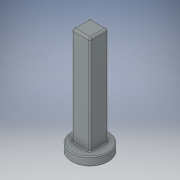
# Autodesk Inventor part: AXp2c
Saved by Autodesk Inventor 2019.3 (Build 233278000, 278)
## iProperties
Company: Unknown
Created: 2018-11-05
Part Number: AXp2c
Material: Generic
Description: Unknown
Document SubType Name: Modeling
Designer: Varga Daniel
Density: 1 g/cm^3
Appearance: Default
Sending System: DEX
Preprocessor: ST-DEVELOPER v16.7
Axle_length: 20,000 mm
Upper_fillet: 0,400 mm
Title: Axeis 2
Author: Unknown
Autodesk Inventor part; units mm, degrees
ref_plane "YZ Plane" through (0, 0, 0) normal (1, 0, 0) x (0, 1, 0)
ref_plane "XZ Plane" through (0, 0, 0) normal (0, 1, 0) x (-1, 0, 0)
ref_plane "XY Plane" through (0, 0, 0) normal (0, 0, 1) x (1, 0, 0)
derived "Connector_pin_base.ipt"
sketch "Pin_base_sketch" plane through (0, 0, 0) normal (0, 0, 1) x (1, 0, 0)
  line L0 (0, 0) -> (23.0918, 0) construction
  line L1 (0, 0) -> (0, 6.22) construction
  line L2 (0, 3.75) -> (0.563, 3.75)
  line L3 (0.863, 3.45) -> (0.863, 2.475)
  line L4 (0.863, 2.475) -> (9.988, 2.475)
  line L5 (9.988, 2.475) -> (9.988, 0)
  line L6 (0, 0) -> (0, 3.75)
  line L7 (0, 0) -> (9.988, 0)
  line L8 (9.288, 2.475) -> (9.288, 2.6)
  line L9 (9.988, 2.475) -> (9.988, 2.4774)
  arc A0 (9.988, 2.4774) -> (9.8454, 2.7031) centre (9.738, 2.4774) ccw
  arc A1 (9.8454, 2.7031) -> (9.288, 2.6) centre (9.6379, 2.267) ccw
  line L10 (9.8454, 2.7031) -> (9.8454, -0.0362) construction
  line L11 (8.9584, 2.75) -> (10.3858, 2.75) construction
  arc A2 (0.863, 3.45) -> (0.563, 3.75) centre (0.563, 3.45) ccw
  line L12 (0.863, 2.475) -> (0.863, 0)
  line L13 (-0.863, 2.475) -> (-0.863, 0)
  line L14 (-0.863, 3.45) -> (-0.863, 2.475)
  arc A3 (-0.563, 3.75) -> (-0.863, 3.45) centre (-0.563, 3.45) ccw
  line L15 (0, 3.75) -> (-0.563, 3.75)
  line L16 (0, 0) -> (-23.0918, 0) construction
  line L17 (0, 0) -> (-9.988, 0)
  line L18 (-0.863, 2.475) -> (-9.988, 2.475)
  line L19 (-9.288, 2.475) -> (-9.288, 2.6)
  arc A4 (-9.288, 2.6) -> (-9.8454, 2.7031) centre (-9.6379, 2.267) ccw
  arc A5 (-9.8454, 2.7031) -> (-9.988, 2.4774) centre (-9.738, 2.4774) ccw
  line L20 (-9.988, 2.475) -> (-9.988, 2.4774)
  line L21 (-8.9584, 2.75) -> (-10.3858, 2.75) construction
  line L22 (-9.8454, 2.7031) -> (-9.8454, -0.0362) construction
  line L23 (-9.988, 2.475) -> (-9.988, 0)
  line L24 (9.638, 3.1946) -> (9.638, -1.2485) construction
derived "Base_part.ipt"
sketch "Axle_sketch" plane through (0, 0, 0) normal (0, 1, 0) x (-1, 0, 0)
  circle A0 centre (-15.8957, 4.3197) radius 2.5 construction
  line L0 (-14.4207, 2.4447) -> (-17.3707, 2.4447)
  line L1 (-17.7707, 2.8447) -> (-17.7707, 5.7947)
  line L2 (-17.3707, 6.1947) -> (-14.4207, 6.1947)
  line L3 (-14.0207, 5.7947) -> (-14.0207, 2.8447)
  line L4 (-14.0207, 2.4447) -> (-17.7707, 6.1947) construction
  line L5 (-17.7707, 2.4447) -> (-14.0207, 6.1947) construction
  arc A1 (-14.4207, 2.4447) -> (-14.0207, 2.8447) centre (-14.4207, 2.8447) ccw
  arc A2 (-17.7707, 2.8447) -> (-17.3707, 2.4447) centre (-17.3707, 2.8447) ccw
  arc A3 (-14.0207, 5.7947) -> (-14.4207, 6.1947) centre (-14.4207, 5.7947) ccw
  arc A4 (-17.3707, 6.1947) -> (-17.7707, 5.7947) centre (-17.3707, 5.7947) ccw
  point P0 (0, 0)
sketch "Sketch1" plane through (0, 0, 0) normal (0, 1, 0) x (-1, 0, 0)
  line L0 (-1.475, -1.875) -> (1.475, -1.875)
  line L1 (1.875, -1.475) -> (1.875, 1.475)
  line L2 (1.475, 1.875) -> (-1.475, 1.875)
  line L3 (-1.875, 1.475) -> (-1.875, -1.475)
  line L4 (-1.875, -1.875) -> (1.875, 1.875) construction
  line L5 (1.875, -1.875) -> (-1.875, 1.875) construction
  arc A0 (-1.875, -1.475) -> (-1.475, -1.875) centre (-1.475, -1.475) ccw
  arc A1 (1.475, -1.875) -> (1.875, -1.475) centre (1.475, -1.475) ccw
  arc A2 (1.875, 1.475) -> (1.475, 1.875) centre (1.475, 1.475) ccw
  arc A3 (-1.475, 1.875) -> (-1.875, 1.475) centre (-1.475, 1.475) ccw
  circle A4 centre (0, 0) radius 2.5 construction
  line L6 (-14.4207, 2.4447) -> (-17.3707, 2.4447) construction
  arc A5 (-14.4207, 2.4447) -> (-14.0207, 2.8447) centre (-14.4207, 2.8447) ccw construction
  line L7 (-14.0207, 5.7947) -> (-14.0207, 2.8447) construction
  circle A6 centre (-15.8957, 4.3197) radius 2.5 construction
  line L8 (-17.3707, 6.1947) -> (-14.4207, 6.1947) construction
  arc A7 (-17.3707, 6.1947) -> (-17.7707, 5.7947) centre (-17.3707, 5.7947) ccw construction
  line L9 (-17.7707, 2.8447) -> (-17.7707, 5.7947) construction
  arc A8 (-17.7707, 2.8447) -> (-17.3707, 2.4447) centre (-17.3707, 2.8447) ccw construction
  arc A9 (-14.0207, 5.7947) -> (-14.4207, 6.1947) centre (-14.4207, 5.7947) ccw construction
  dimension "d0" = 3.75
  dimension "d1" = 3.75
  dimension "d2" = 0.4
  dimension "d11" = 5
  dimension "d13" = 3.75
  dimension "d14" = 0.4
  constraints: 12 end point, 8 point on circle, 8 point on line, 8 tangent, 5 centre point, 3 equal radius, 2 midpoint, 2 parallel, 1 coincident, 1 horizontal, 1 perpendicular
  measures "d0" distance of L4.end L5.end
  measures "d1" distance between parallel lines of L2 L0
  measures "d2" radius of A0
  measures "d11" diameter of A4
  measures "d13" distance between parallel lines of L7 L9
  measures "d14" radius of A8
extrude "Extrusion4" add sketch "Sketch1" along normal blind 20
fillet "Fillet2" radius 0.4 8 edges at (1.7578, 20, -1.7578) (0, 20, -1.875) (-1.7578, 20, -1.7578) (-1.875, 20, 0) (-1.7578, 20, 1.7578) (0, 20, 1.875) (1.7578, 20, 1.7578) (1.875, 20, 0)
ref_plane "Work Plane3" through (-1.475, 0, 0) normal (0, 0, 1) x (1, 0, 0)
ref_plane "Work Plane4" through (0, 0, -1.475) normal (-1, 0, 0) x (0, 0, 1)
sketch "Sketch6" plane through (0, 0, 0) normal (0, 0, 1) x (1, 0, 0)
  line L0 (0.863, 2.475) -> (0.863, 0) construction
  line L1 (0.863, 3.45) -> (0.863, 2.475) construction
  arc A0 (0.863, 3.45) -> (0.563, 3.75) centre (0.563, 3.45) ccw construction
  line L2 (0, 3.75) -> (0.563, 3.75) construction
  line L3 (0, 0) -> (0, 6.22) construction
  line L4 (0, 0) -> (23.0918, 0) construction
  line L5 (-1.475, 0) -> (1.475, 0) construction
  line L6 (-1.875, 0) -> (-1.875, 19.6) construction
  line L7 (1.875, 0) -> (1.875, 19.6) construction
  line L8 (1.475, 0) -> (-1.475, 0) construction
  line L9 (1.875, 0) -> (1.475, 0) construction
  line L10 (1.475, 0) -> (1.875, 0) construction
  line L11 (-1.475, 0) -> (1.475, 0) construction
  line L12 (-1.875, 0) -> (-1.475, 0) construction
  line L13 (-1.475, 0) -> (-1.875, 0) construction
  line L14 (0, 0) -> (0, -2.3465) construction
  line L15 (0, 24.4693) -> (0, -6.8158) construction
  line L16 (0, 0) -> (3.55, 0)
  line L17 (0, -1.8) -> (3.55, -1.8)
  line L18 (3.75, -1.6) -> (3.75, -0.2)
  arc A1 (3.75, -0.2) -> (3.55, 0) centre (3.55, -0.2) ccw
  arc A2 (3.55, -1.8) -> (3.75, -1.6) centre (3.55, -1.6) ccw
  line L19 (0, -1.8) -> (0, 0)
  dimension "d19" = 7.5
  dimension "d20" = 0.3
  dimension "d21" = 7.5
  dimension "d23" = 1.8
  dimension "d24" = 0.2
  dimension "d25" = 0.2
  constraints: 10 end point, 4 point on circle, 4 tangent, 2 centre point, 2 collinear, 2 point on line, 1 horizontal, 1 perpendicular
  measures "d19" diameter of L2 L4
  measures "d20" radius of A0
  measures "d21" diameter of L18 L14
  measures "d23" distance between parallel lines of L17 L16
  measures "d24" radius of A1
  measures "d25" radius of A2
revolve "Revolution1" add sketch "Sketch6" angle 360 about axis through (0, 0, 0) along (0, 1, 0)
fillet "Fillet3" radius 0.2 8 edges at (1.7578, 0, 1.7578) (1.875, 0, 0) (1.7578, 0, -1.7578) (0, 0, -1.875) (-1.7578, 0, -1.7578) (-1.875, 0, 0) (-1.7578, 0, 1.7578) (0, 0, 1.875)
sketch "Sketch7" plane through (1.875, 19.6, 1.475) normal (1, 0, 0) x (0, 0, -1)
  line L0 (2.95, -19.4) -> (0, -19.4) projected
  line L1 (2.95, -19.4) -> (2.95, 0) projected
  line L2 (0, 0) -> (2.95, 0) projected
  line L3 (0, -19.4) -> (0, 0) projected
  line L4 (12.95, 10) -> (12.95, -29.4)
  line L5 (12.95, -29.4) -> (-10, -29.4)
  line L6 (-10, -29.4) -> (-10, 10)
  line L7 (-10, 10) -> (12.95, 10)
  point P0 (1.475, -19.6)
  dimension "d28" = 10
  constraints: 8 end point, 3 other
  measures "d28" distance between parallel lines of L1 L4
extrude "Printable_extrusion" [suppressed]
equation "\"d0\" = d13"
equation "\"d1\" = d0"
equation "\"d2\" = d14"
equation "\"d15\" = Axle_length"
equation "\"d17\" = Upper_fillet"
equation "\"d21\" = d19"
equation "\"d23\" = Axle_collar_thickness"
equation "\"d24\" = Axle_collar_fillet"
equation "\"d25\" = d24"
equation "\"d27\" = Axle_collar_fillet"
equation "\"Axle_length\" = 20"
equation "\"Upper_fillet\" = 0.4"
equation "\"Axle_collar_fillet\" = 0.2"
equation "\"Axle_collar_thickness\" = 1.8"
body "Solid1"
